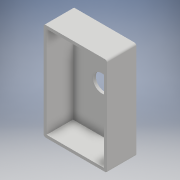
# Autodesk Inventor part: NadstavbaArduinoHranata
Saved by Autodesk Inventor 2017 (Build 210142000, 142)
## iProperties
Created: 2019-02-06
Part Number: NadstavbaArduinoHranata
Material: Generic
Document SubType Name: Modeling
Designer: Denis Kurka
Density: 1 g/cm^3
Appearance: Default
Author: Denis Kurka
Autodesk Inventor part; units mm, degrees
ref_plane "YZ Plane" through (0, 0, 0) normal (1, 0, 0) x (0, 1, 0)
ref_plane "XZ Plane" through (0, 0, 0) normal (0, 1, 0) x (-1, 0, 0)
ref_plane "XY Plane" through (0, 0, 0) normal (0, 0, 1) x (1, 0, 0)
sketch "Sketch1" plane through (0, 0, 0) normal (0, 1, 0) x (-1, 0, 0)
  line L0 (0, 0) -> (65, 0)
  line L1 (65, 0) -> (65, -100)
  line L2 (65, -100) -> (0, -100)
  line L3 (0, -100) -> (0, 0)
  line L4 (62, -3) -> (3, -3)
  line L5 (3, -3) -> (3, -97)
  line L6 (3, -97) -> (62, -97)
  line L7 (62, -97) -> (62, -3)
  dimension "d0" = 100
  dimension "d1" = 65
  dimension "d2" = 3
  dimension "d3" = 3
  dimension "d5" = 3
  dimension "d6" = 3
  constraints: 16 end point, 4 parallel, 2 horizontal, 2 perpendicular
  measures "d0" distance of L0.end L1.end
  measures "d1" distance of L1.end L2.end
  measures "d2" distance between parallel lines of L1 L7
  measures "d3" distance between parallel lines of L2 L6
  measures "d5" distance between parallel lines of L0 L4
  measures "d6" distance between parallel lines of L3 L5
extrude "Extrusion1" add sketch "Sketch1" along normal blind 30
sketch "Sketch2" plane through (-62, 0, -97) normal (0, 0, 1) x (1, 0, 0)
  line L0 (62, 30) -> (-3, 30) projected
  line L1 (-3, 0) -> (-3, 30) projected
  line L2 (62, 30) -> (-3, 30)
  line L3 (-3, 30) -> (-3, 27)
  line L4 (-3, 27) -> (62, 27)
  line L5 (62, 27) -> (62, 30)
  point P0 (62, 0)
  dimension "d9" = 3
  constraints: 8 end point, 2 parallel, 1 horizontal, 1 perpendicular, 1 point on line
  measures "d9" distance between parallel lines of L0 L4
extrude "Extrusion2" add sketch "Sketch2" along normal blind 97
sketch "Sketch3" plane through (0, 30, 0) normal (0, 1, 0) x (1, 0, 0)
  circle A0 centre (-32.5, 50) radius 9
  line L0 (-65, 100) -> (-65, 0) projected
  line L1 (0, 0) -> (0, 100) projected
  line L2 (-65, 0) -> (0, 0) projected
  line L3 (0, 100) -> (-65, 100) projected
  dimension "d12" = 18
  dimension "d14" = 32.5
  dimension "d15" = 32.5
  dimension "d16" = 50
  dimension "d17" = 50
  constraints: 1 centre point
  measures "d12" diameter of A0
  measures "d14" distance from line of L0 A0.centre
  measures "d15" distance from line of L1 A0.centre
  measures "d16" distance from line of L2 A0.centre
  measures "d17" distance from line of L3 A0.centre
extrude "Extrusion3" cut sketch "Sketch3" against normal blind 97 contours A0
fillet "Fillet1" radius 2 4 edges at (0, 15, 0) (-65, 15, 0) (0, 15, -100) (-65, 15, -100)
equation "\"d14\" = d15"
equation "\"d16\" = d17"
body "Solid1"
